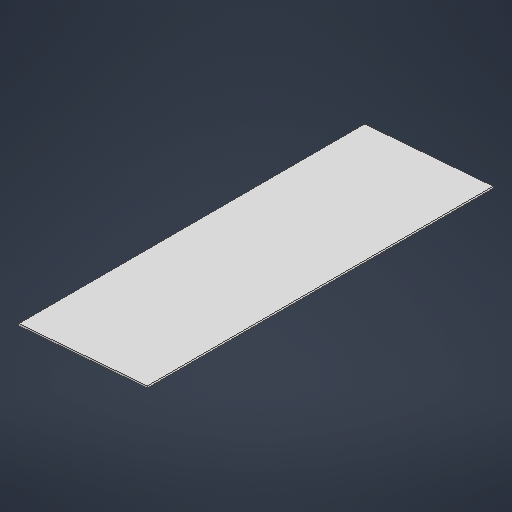
# Autodesk Inventor part: d
Saved by Autodesk Inventor 2027 (Build 310192000, 192)
## iProperties
Created: 2026-02-05
Part Number: d
Material: Generic
Document SubType Name: Modeling
Designer: Joefi
Density: 1 g/cm^3
Appearance: Default
Author: Joefi
Autodesk Inventor part; units mm, degrees
ref_plane "YZ Plane" through (0, 0, 0) normal (1, 0, 0) x (0, 1, 0)
ref_plane "XZ Plane" through (0, 0, 0) normal (0, 1, 0) x (-1, 0, 0)
ref_plane "XY Plane" through (0, 0, 0) normal (0, 0, 1) x (1, 0, 0)
sketch "Sketch1" plane through (0, 0, 0) normal (0, 1, 0) x (-1, 0, 0)
  line L0 (-6.5173, 34.655) -> (5.399, 35.6975)
  arc A0 (10.8348, 30.7166) -> (5.399, 35.6975) centre (5.8348, 30.7166) ccw
  line L1 (10.8348, 30.7166) -> (10.8348, -31.0313)
  arc A1 (6.2705, -36.0123) -> (10.8348, -31.0313) centre (5.8348, -31.0313) ccw
  line L2 (6.2705, -36.0123) -> (-5.6458, -37.0548)
  arc A2 (-11.0815, -32.0739) -> (-5.6458, -37.0548) centre (-6.0815, -32.0739) ccw
  line L3 (-11.0815, -32.0739) -> (-11.0815, 29.674)
  arc A3 (-6.5173, 34.655) -> (-11.0815, 29.674) centre (-6.0815, 29.674) ccw
  line L4 (12.8348, 38.3557) -> (-13.0815, 36.0883)
  line L5 (-13.0815, 36.0883) -> (-13.0815, -39.713)
  line L6 (-13.0815, -39.713) -> (12.8348, -37.4456)
  line L7 (12.8348, -37.4456) -> (12.8348, 38.3557)
  line L8 (12.6348, 38.1375) -> (-12.8815, 35.9051)
  line L9 (-12.8815, 35.9051) -> (-12.8815, -39.4948)
  line L10 (-12.8815, -39.4948) -> (12.6348, -37.2624)
  line L11 (12.6348, -37.2624) -> (12.6348, 38.1375)
  point P0 (0, 0)
  dimension "d0" = 0.2
  constraints: 24 end point, 8 point on circle, 4 centre point, 3 other
  measures "d0" distance between parallel lines of L7 L11
extrude "Extrusion1" add sketch "Sketch1" along normal blind 0.4 contours L0 A0 L1 A1 L2 A2 L3 A3 | L7 L6 L5 L4 | L11 L10 L9 L8
body "Solid1"
